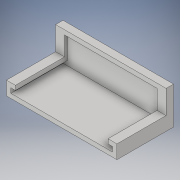
# Autodesk Inventor part: креплениедлякамерыверх
Saved by Autodesk Inventor 2019 (Build 230136000, 136)
## iProperties
Created: 2020-01-23
Part Number: креплениедлякамерыверх
Material: Типовые
Document SubType Name: Modeling
Designer: UlyaKZ
Density: 1 g/cm^3
Appearance: По умолчанию
Author: UlyaKZ
Autodesk Inventor part; units mm, degrees
ref_plane "YZ Plane" through (0, 0, 0) normal (1, 0, 0) x (0, 1, 0)
ref_plane "XZ Plane" through (0, 0, 0) normal (0, 1, 0) x (-1, 0, 0)
ref_plane "XY Plane" through (0, 0, 0) normal (0, 0, 1) x (1, 0, 0)
sketch "Эскиз1" plane through (0, 0, 0) normal (0, 0, 1) x (1, 0, 0)
  line L0 (0, 0) -> (74.2, 0)
  line L1 (0, 0) -> (0, 9.2)
  line L2 (0, 9.2) -> (6, 9.2)
  line L3 (6, 9.2) -> (6, 6.2)
  line L4 (6, 6.2) -> (3, 6.2)
  line L5 (3, 6.2) -> (3, 3)
  line L6 (71.2, 3) -> (71.2, 6.2)
  line L7 (71.2, 6.2) -> (68.2, 6.2)
  line L8 (68.2, 6.2) -> (68.2, 9.2)
  line L9 (68.2, 9.2) -> (74.2, 9.2)
  line L10 (74.2, 9.2) -> (74.2, 0)
  line L11 (3, 3) -> (71.2, 3)
  dimension "d2" = 68.2
  dimension "d3" = 3
  dimension "d4" = 3
  dimension "d5" = 3
  dimension "d6" = 3
  dimension "d7" = 3
  dimension "d8" = 3
  dimension "d9" = 3
  dimension "d10" = 3.2
  constraints: 24 end point, 6 perpendicular, 2 point on line, 2 vertical, 2 vertical alignment, 1 horizontal, 1 horizontal alignment, 1 parallel
  measures "d2" distance between parallel lines of L5 L6
  measures "d3" distance between parallel lines of L6 L10
  measures "d4" distance between parallel lines of L1 L5
  measures "d5" distance between parallel lines of L0 L11
  measures "d6" distance of L6.end L7.end
  measures "d7" distance of L3.end L4.end
  measures "d8" distance of L7.end L8.end
  measures "d9" distance of L2.end L3.end
  measures "d10" distance between parallel lines of L11 L7
extrude "Выдавливание1" add sketch "Эскиз1" along normal blind 35
sketch "Эскиз2" plane through (0, 0, 0) normal (0, -1, 0) x (1, 0, 0)
  line L0 (6, 0) -> (0, 0) projected
  line L1 (0, 0) -> (74.2, 0)
  line L2 (74.2, 0) -> (74.2, -3)
  line L3 (74.2, -3) -> (0, -3)
  line L4 (0, -3) -> (0, 0)
  point P0 (74.2, -1.5)
  dimension "d13" = 3
  constraints: 8 end point, 3 perpendicular, 1 horizontal, 1 midpoint, 1 vertical alignment
  measures "d13" distance between parallel lines of L1 L3
extrude "Выдавливание2" add sketch "Эскиз2" against normal blind 25
sketch "Эскиз3" plane through (0, 25, 0) normal (0, 0, 1) x (1, 0, 0)
  line L0 (74.2, -15.8) -> (74.2, 0) projected
  line L1 (74.2, -15.8) -> (74.2, 0)
  line L2 (0, 0) -> (74.2, 0) projected
  line L3 (74.2, 0) -> (0, 0)
  line L4 (6, -15.8) -> (0, -15.8) projected
  line L5 (0, 0) -> (0, -15.8)
  line L6 (0, -15.8) -> (6, -15.8)
  line L7 (6, -15.8) -> (6, -3)
  line L8 (6, -3) -> (68.2, -3)
  line L9 (68.2, -3) -> (68.2, -15.8)
  line L10 (74.2, -15.8) -> (68.2, -15.8) projected
  line L11 (74.2, -15.8) -> (68.2, -15.8)
  point P0 (0, -25)
  dimension "d16" = 3
  constraints: 16 end point, 5 perpendicular, 1 coincident, 1 collinear, 1 horizontal, 1 vertical
  measures "d16" distance between parallel lines of L8 L2
extrude "Выдавливание3" add sketch "Эскиз3" along normal blind 2
